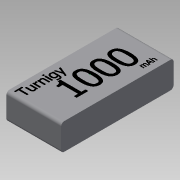
# Autodesk Inventor part: Baterai 1.0
Saved by Autodesk Inventor 2015 SP1 (Build 190203100, 203)
## iProperties
Created: 2015-03-25
Part Number: Baterai 1.0
Material: Generic
Document SubType Name: Modeling
Designer: Rafi Kurnia Putra
Density: 1 g/cm^3
Appearance: Default
Author: Rafi Kurnia Putra
Autodesk Inventor part; units mm, degrees
ref_plane "YZ Plane" through (0, 0, 0) normal (1, 0, 0) x (0, 1, 0)
ref_plane "XZ Plane" through (0, 0, 0) normal (0, 1, 0) x (-1, 0, 0)
ref_plane "XY Plane" through (0, 0, 0) normal (0, 0, 1) x (1, 0, 0)
sketch "Sketch1" plane through (0, 0, 0) normal (0, 0, 1) x (1, 0, 0)
  line L0 (-17.5, -36) -> (17.5, -36)
  line L1 (17.5, -36) -> (17.5, 36)
  line L2 (17.5, 36) -> (-17.5, 36)
  line L3 (-17.5, 36) -> (-17.5, -36)
  line L4 (-17.5, -36) -> (17.5, 36) construction
  line L5 (17.5, -36) -> (-17.5, 36) construction
  point P0 (0, 0)
  dimension "d0" = 35
  dimension "d1" = 72
  constraints: 12 end point, 2 midpoint, 2 parallel, 1 horizontal, 1 perpendicular
  measures "d0" distance of L2.end L1.end
  measures "d1" distance of L1.end L0.end
extrude "Extrusion1" add sketch "Sketch1" along normal blind 17
fillet "Fillet1" radius 2 4 edges at (0, 36, 17) (0, 36, 0) (0, -36, 0) (0, -36, 17)
sketch "Sketch3" plane through (0, 0, 17) normal (0, 0, 1) x (1, 0, 0)
  line L0 (-6.9109, -19.3056) -> (-6.9109, -0.1322) construction
  line L1 (-6.9109, -0.1322) -> (3.5024, -0.1322) construction
  line L2 (3.5024, -0.1322) -> (3.5024, -19.3056) construction
  line L3 (3.5024, -19.3056) -> (-6.9109, -19.3056) construction
  line L4 (9.9359, 20.457) -> (9.9359, 30.0692) construction
  line L5 (9.9359, 30.0692) -> (13.5919, 30.0692) construction
  line L6 (13.5919, 30.0692) -> (13.5919, 20.457) construction
  line L7 (13.5919, 20.457) -> (9.9359, 20.457) construction
  line L8 (-15.0335, -33.4145) -> (-15.0335, -5.4059) construction
  line L9 (-15.0335, -5.4059) -> (-7.1638, -5.4059) construction
  line L10 (-7.1638, -5.4059) -> (-7.1638, -33.4145) construction
  line L11 (-7.1638, -33.4145) -> (-15.0335, -33.4145) construction
  point P0 (0, 0)
  constraints: 6 other
body "Solid1"
